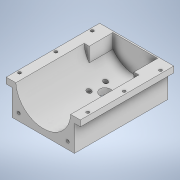
# Autodesk Inventor part: engine_sleeve_up
Saved by Autodesk Inventor 2020.1 (Build 241239000, 239)
## iProperties
Created: 2022-02-06
Part Number: engine_sleeve_up
Material: Generic
Document SubType Name: Modeling
Designer: OEM
Density: 1 g/cm^3
Appearance: Default
Author: OEM
Autodesk Inventor part; units mm, degrees
ref_plane "YZ Plane" through (0, 0, 0) normal (1, 0, 0) x (0, 1, 0)
ref_plane "XZ Plane" through (0, 0, 0) normal (0, 1, 0) x (-1, 0, 0)
ref_plane "XY Plane" through (0, 0, 0) normal (0, 0, 1) x (1, 0, 0)
sketch "Sketch1" plane through (0, 0, 0) normal (0, 1, 0) x (-1, 0, 0)
  circle A0 centre (0, 0) radius 11 construction
  circle A1 centre (0, 0) radius 3.75
  circle A2 centre (0, 0) radius 7.875 construction
  line L0 (16.292, 0) -> (-19, 0) construction
  line L1 (0, 21) -> (0, -27.3544) construction
  line L2 (0, -21) -> (21, -21)
  line L3 (0, -21) -> (-21, -21)
  line L4 (0, 0) -> (21, -21) construction
  circle A3 centre (5.5685, -5.5685) radius 0.75
  circle A4 centre (-5.5685, -5.5685) radius 0.75
  circle A5 centre (5.5685, 5.5685) radius 0.75
  circle A6 centre (-5.5685, 5.5685) radius 0.75
  line L5 (-25, -21) -> (-21, -21)
  line L6 (25, -21) -> (21, -21)
  circle A7 centre (23, -14) radius 1
  circle A8 centre (-23, -14) radius 1
  line L7 (-25, 42) -> (25, 42)
  line L8 (25, -21) -> (25, 42)
  line L9 (21, -21) -> (21, 42)
  line L10 (-21, -21) -> (-21, 42)
  line L11 (-25, -21) -> (-25, 42)
  line L12 (25, 10.5) -> (-25, 10.5) construction
  circle A9 centre (23, 35) radius 1
  circle A10 centre (-23, 35) radius 1
  circle A11 centre (23, 10.5) radius 1
  circle A12 centre (-23, 10.5) radius 1
  circle A13 centre (5.5685, 5.5685) radius 1.5
  circle A14 centre (5.5685, -5.5685) radius 1.5
  circle A15 centre (-5.5685, 5.5685) radius 1.5
  circle A16 centre (-5.5685, -5.5685) radius 1.5
  dimension "d8" = 15.75
  dimension "d2" = 7.5
  dimension "d4" = 22
  dimension "d17" = 21
  dimension "d26" = 1.5
  dimension "d38" = 63
  dimension "d39" = 21
  dimension "d40" = 2
  dimension "d41" = 2
  dimension "d53" = 3
  dimension "d106" = 4
  dimension "d107" = 7
  constraints: 26 end point, 16 centre point, 11 symmetric about line, 5 perpendicular, 5 point on line, 2 coincident, 2 midpoint, 1 horizontal, 1 parallel, 1 vertical, 13 other
  measures "d2" diameter of A1
  measures "d4" diameter of A0
  measures "d17" distance from line of point (0, 0) L2
  measures "d26" diameter of A3
  measures "d38" distance of L6.start L7.end
  measures "d39" distance of L2.start L2.end
  measures "d40" diameter of A9
  measures "d41" diameter of A11
  measures "d53" diameter of A13
  measures "d106" distance of L6.start L2.end
  measures "d107" distance from line of L7 A9.centre
extrude "Extrusion9" add sketch "Sketch1" along normal blind 45 contours A1 | L3 L10 L7 L9 L2 | A3 | A4 | A5 | A6 | A13 | A14 | A15 | A16
extrude "Extrusion10" add sketch "Sketch1" along normal blind 27.5 contours L9 L7 L8 L6 | L5 L11 L7 L10
extrude "Extrusion11" cut sketch "Sketch1" along normal blind 17.5 contours L9 L7 L8 L6 | L5 L11 L7 L10
extrude "Extrusion13" cut sketch "Sketch1" along normal blind 6 contours A1 | A3 | A4 | A5 | A6 | A13 | A14 | A15 | A16
extrude "Extrusion15" add sketch "Sketch1" along normal blind 3.5 contours A13 | A14 | A15 | A16
sketch "Sketch5" plane through (-21, 45, 42) normal (0, 0, 1) x (1, 0, 0)
  line L0 (0, -45) -> (42, -45) construction
  line L1 (0, -17.5) -> (0, 0) construction
  line L2 (42, -45) -> (0, -45) construction
  line L3 (0, -45) -> (0, 0) construction
  line L4 (0, 0) -> (42, 0) construction
  line L5 (42, 0) -> (42, -45) construction
  line L6 (42, 0) -> (0, -45) construction
  line L7 (0, 0) -> (42, 0) construction
  line L8 (0, 0.0001) -> (42, -44.9999) construction
  circle A0 centre (21, -22.4999) radius 18.5
  line L9 (10.2856, -7.4184) -> (31.7144, -7.4184)
  line L10 (5.9185, -11.7855) -> (5.9185, -33.2143)
  line L11 (36.0815, -11.7855) -> (36.0815, -33.2143)
  circle A1 centre (21, -22.4999) radius 13.5 construction
  line L12 (34.0815, -9.4184) -> (7.9185, -35.5814) construction
  line L13 (21, -45) -> (21, 0.5001) construction
  line L14 (7.9185, -9.4184) -> (34.0815, -35.5814) construction
  line L15 (7.9185, -9.4184) -> (34.0815, -9.4184) construction
  line L16 (7.9185, -9.4184) -> (7.9185, -35.5814) construction
  line L17 (34.0815, -35.5814) -> (34.0815, -9.4184) construction
  circle A2 centre (4.5, -40.1786) radius 1
  circle A3 centre (37.5, -40.1786) radius 1
  circle A4 centre (4.5, -4.8214) radius 1
  circle A5 centre (37.5, -4.8214) radius 1
  line L18 (47, -22.4999) -> (47, -23.4999)
  line L19 (47, -22.4999) -> (-3.9988, -22.4999) construction
  line L20 (47, -23.4999) -> (42, -23.4999)
  line L21 (42, -23.4999) -> (39.473, -23.4999)
  line L22 (39.473, -23.4999) -> (36.0815, -23.4999)
  line L23 (36.0815, -23.4999) -> (21, -23.4999)
  line L24 (-5, -23.4999) -> (0, -23.4999)
  line L25 (0, -23.4999) -> (2.527, -23.4999)
  line L26 (2.527, -23.4999) -> (5.9185, -23.4999)
  line L27 (5.9185, -23.4999) -> (21, -23.4999)
  line L28 (-5, -22.4999) -> (-5, -23.4999)
  line L29 (47, -22.4999) -> (47, -21.4999)
  line L30 (47, -21.4999) -> (42, -21.4999)
  line L31 (42, -21.4999) -> (39.473, -21.4999)
  line L32 (39.473, -21.4999) -> (36.0815, -21.4999)
  line L33 (36.0815, -21.4999) -> (21, -21.4999)
  line L34 (-5, -21.4999) -> (0, -21.4999)
  line L35 (0, -21.4999) -> (2.527, -21.4999)
  line L36 (2.527, -21.4999) -> (5.9185, -21.4999)
  line L37 (5.9185, -21.4999) -> (21, -21.4999)
  line L38 (-5, -22.4999) -> (-5, -21.4999)
  line L39 (21, 0.5001) -> (42, 0.5001)
  line L40 (42, 0.5001) -> (47, 0.5001)
  line L41 (47, 0.5001) -> (47, -21.4999)
  line L42 (21, 0.5001) -> (0, 0.5001)
  line L43 (0, 0.5001) -> (-5, 0.5001)
  line L44 (-5, 0.5001) -> (-5, -21.4999)
  line L45 (21, -45.4999) -> (42, -45.4999)
  line L46 (42, -45.4999) -> (47, -45.4999)
  line L47 (47, -45.4999) -> (47, -23.4999)
  line L48 (-5, -45.4999) -> (-5, -23.4999)
  line L49 (0, -45.4999) -> (-5, -45.4999)
  line L50 (21, -45.4999) -> (0, -45.4999)
  point P0 (39.5, -22.4999)
  dimension "d58" = 37
  dimension "d70" = 27
  dimension "d73" = 2
  dimension "d74" = 45
  dimension "d75" = 2
  dimension "d76" = 2
  dimension "d77" = 42
  dimension "d79" = 2
  dimension "d80" = 4.5
  dimension "d89" = 1
  dimension "d90" = 1
  dimension "d105" = 23
  constraints: 96 end point, 23 symmetric about line, 13 point on line, 5 centre point, 5 perpendicular, 4 horizontal, 3 horizontal alignment, 2 parallel, 2 vertical alignment, 1 coincident, 1 midpoint, 1 vertical, 13 other
  measures "d70" diameter of A1
  measures "d73" distance between parallel lines of L17 L11
  measures "d74" angle of L13 L12
  measures "d75" distance between parallel lines of L9 L15
  measures "d76" distance between parallel lines of L16 L10
  measures "d77" distance of L0.start L0.end
  measures "d79" diameter of A2
  measures "d80" distance from line of L3 A2.centre
  measures "d89" distance of L23.end point (21, -22.5)
  measures "d90" distance of L37.end point (21, -22.5)
  measures "d105" distance of A1.centre L13.end
extrude "Extrusion16" cut sketch "Sketch5" against normal blind 62 contours L11 L33 L37 L10 A0 L9 | L11 L23 L27 L10 L37 L33 | A0 L10 L27 L23 L11
extrude "Extrusion18" cut sketch "Sketch5" against normal blind 46 contours A0 L22 L11 L32 | L32 L11 A0 | A0 L11 L22 | L9 A0 | A0 L26 L10 | L36 A0 L10 | L10 L26 A0 L36
extrude "Extrusion19" cut sketch "Sketch5" against normal blind 5 contours A2 | A3 | A4 | A5
extrude "Extrusion23" cut sketch "Sketch5" against normal blind 70 contours A0 L22 L11 L32 | A0 L31 L30 L29 L18 L20 L21 | L32 L11 A0 | A0 L35 L34 L44 L43 L42 L39 L40 L41 L30 L31 | L11 L33 L37 L10 A0 L9 | L11 L23 L27 L10 L37 L33 | L9 A0 | L36 A0 L10 | L10 L26 A0 L36 | L25 L24 L28 L38 L34 L35 A0 | A4 | A5
equation "\"d41\" = d40"
body "Solid2"
